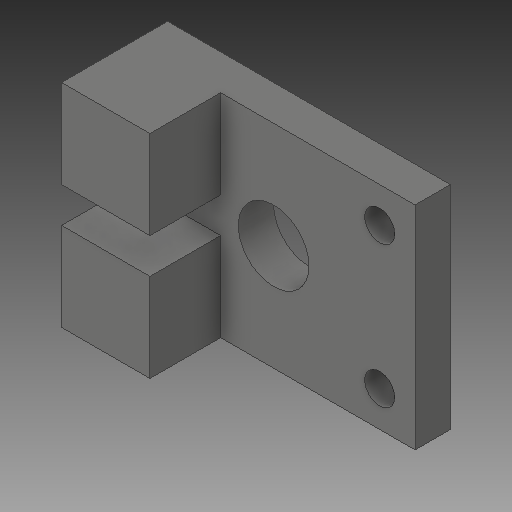
# Autodesk Inventor part: YCartBeltClamp
Saved by Autodesk Inventor 2019 (Build 230136000, 136)
## iProperties
Created: 2019-09-07
Part Number: YCartBeltClamp
Material: Generic
Document SubType Name: Modeling
Designer: Bruno
Density: 1 g/cm^3
Appearance: Default
Mass: 8.59044 g
Surface Area: 41.7677 cm^2
Volume: 8.59044 cm^3
Author: Bruno
## iProperties of the stored document YCartBeltClamp_3DPrint.ipt
Created: 2019-09-09
Part Number: YCartBeltClamp_3DPrint
Material: Generic
Document SubType Name: Modeling
Designer: Bruno
Density: 1 g/cm^3
Appearance: Default
Author: Bruno
Autodesk Inventor part; units mm, degrees
ref_plane "YZ Plane" through (0, 0, 0) normal (1, 0, 0) x (0, 1, 0)
ref_plane "XZ Plane" through (0, 0, 0) normal (0, 1, 0) x (-1, 0, 0)
ref_plane "XY Plane" through (0, 0, 0) normal (0, 0, 1) x (1, 0, 0)
sketch "Sketch1" plane through (0, 0, 0) normal (0, 0, 1) x (1, 0, 0)
  line L0 (20, 15) -> (-20, 15)
  line L1 (-20, 15) -> (-20, -15)
  line L2 (-20, -15) -> (20, -15)
  line L3 (20, -15) -> (20, 15)
  line L4 (0, 0) -> (1.9807, 0) construction
  line L5 (0, 0) -> (0, -2.0582) construction
  circle A0 centre (15, -10) radius 2.125 projected
  circle A1 centre (15, 10) radius 2.125 projected
  circle A2 centre (0, 0) radius 2.125 projected
  circle A3 centre (15, -10) radius 2.125
  circle A4 centre (15, 10) radius 2.125
  circle A5 centre (0, 0) radius 2.125
  circle A6 centre (0, 0) radius 2.125 projected
  circle A7 centre (0, 0) radius 5
  dimension "d4" = 40
  dimension "d5" = 30
  dimension "d8" = 10
  constraints: 12 end point, 4 centre point, 4 coincident, 2 concentric, 2 horizontal, 2 parallel, 1 perpendicular, 1 vertical, 2 other
  measures "d4" distance of L0.start L0.end
  measures "d5" distance of L2.end L0.start
  measures "d8" diameter of A7
extrude "Extrusion1" add sketch "Sketch1" along normal blind 5 contours L3 L2 L1 L0
sketch "Sketch3" plane through (0, 0, 5) normal (0, 0, 1) x (1, 0, 0)
  line L0 (-20, -15) -> (20, -15) projected
  line L1 (20, -15) -> (20, 15) projected
  line L2 (20, 15) -> (-20, 15) projected
  line L3 (-7.5, -15) -> (-7.5, -2.5)
  line L4 (-7.5, -2.5) -> (-20, -2.5)
  line L5 (-20, 15) -> (-20, -15) projected
  line L6 (-20, 2.5) -> (-7.5, 2.5)
  line L7 (-7.5, 2.5) -> (-7.5, 15)
  point P0 (0, 0)
  dimension "d9" = 5
  constraints: 8 end point, 6 point on line, 2 equal length, 1 parallel, 1 perpendicular, 1 vertical
  measures "d9" distance between parallel lines of L6 L4
extrude "Extrusion2" add sketch "Sketch3" along normal blind 10 contours L5 L4 L3 L0 | L5 L2 L7 L6
body "Solid1"
